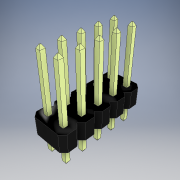
# Autodesk Inventor part: PinHeader-2x5-Male-NoCover
Saved by Autodesk Inventor 2018 (Build 220112000, 112)
## iProperties
Created: 2020-04-19
Part Number: PinHeader-2x5-Male-NoCover
Material: Všeobecné
Document SubType Name: Modeling
Designer: Jozko Mrkvicka
Density: 1 g/cm^3
Appearance: Výchozí
Author: Jozko Mrkvicka
Autodesk Inventor part; units mm, degrees
ref_plane "YZ Plane" through (0, 0, 0) normal (1, 0, 0) x (0, 1, 0)
ref_plane "XZ Plane" through (0, 0, 0) normal (0, 1, 0) x (-1, 0, 0)
ref_plane "XY Plane" through (0, 0, 0) normal (0, 0, 1) x (1, 0, 0)
sketch "Náčrt1" plane through (0, 0, 0) normal (0, 1, 0) x (-1, 0, 0)
  line L0 (0.635, 0) -> (4.445, 0)
  line L1 (4.445, -12.7) -> (0.635, -12.7)
  line L2 (0, -1.905) -> (0.635, -2.54)
  line L3 (0.635, -2.54) -> (0, -3.175)
  line L4 (0, -4.445) -> (0.635, -5.08)
  line L5 (0.635, -5.08) -> (0, -5.715)
  line L6 (0, -6.985) -> (0.635, -7.62)
  line L7 (0.635, -7.62) -> (0, -8.255)
  line L8 (0, -9.525) -> (0.635, -10.16)
  line L9 (0.635, -10.16) -> (0, -10.795)
  line L10 (0, -10.795) -> (0, -12.065)
  line L11 (0, -12.065) -> (0.635, -12.7)
  line L12 (0, -0.635) -> (0.635, 0)
  line L13 (4.445, 0) -> (5.08, -0.635)
  line L14 (5.08, -1.905) -> (4.445, -2.54)
  line L15 (4.445, -2.54) -> (5.08, -3.175)
  line L16 (5.08, -4.445) -> (4.445, -5.08)
  line L17 (4.445, -5.08) -> (5.08, -5.715)
  line L18 (5.08, -6.985) -> (4.445, -7.62)
  line L19 (4.445, -7.62) -> (5.08, -8.255)
  line L20 (5.08, -9.525) -> (4.445, -10.16)
  line L21 (4.445, -10.16) -> (5.08, -10.795)
  line L22 (5.08, -12.065) -> (4.445, -12.7)
  line L23 (0, -1.905) -> (0, -0.635)
  line L24 (0, -4.445) -> (0, -3.175)
  line L25 (0, -6.985) -> (0, -5.715)
  line L26 (0, -12.065) -> (0, -10.795)
  line L27 (0, -9.525) -> (0, -8.255)
  line L28 (5.08, -10.795) -> (5.08, -12.065)
  line L29 (5.08, -8.255) -> (5.08, -9.525)
  line L30 (5.08, -5.715) -> (5.08, -6.985)
  line L31 (5.08, -0.635) -> (5.08, -1.905)
  line L32 (5.08, -3.175) -> (5.08, -4.445)
  point P0 (0, 0)
  constraints: 66 end point, 26 parallel, 21 perpendicular, 1 horizontal
extrude "Vysunutí1" add sketch "Náčrt1" along normal blind 2.54
sketch "Náčrt2" plane through (0, 2.54, 0) normal (0, 1, 0) x (1, 0, 0)
  line L0 (-1.5875, 4.1275) -> (-1.5875, 3.4925)
  line L1 (-1.5875, 3.4925) -> (-0.9525, 3.4925)
  line L2 (-0.9525, 3.4925) -> (-0.9525, 4.1275)
  line L3 (-0.9525, 4.1275) -> (-1.5875, 4.1275)
  line L4 (-4.1275, 4.1275) -> (-4.1275, 3.4925)
  line L5 (-4.1275, 3.4925) -> (-3.4925, 3.4925)
  line L6 (-3.4925, 3.4925) -> (-3.4925, 4.1275)
  line L7 (-3.4925, 4.1275) -> (-4.1275, 4.1275)
  line L8 (-1.5875, 6.6675) -> (-1.5875, 6.0325)
  line L9 (-1.5875, 6.0325) -> (-0.9525, 6.0325)
  line L10 (-0.9525, 6.0325) -> (-0.9525, 6.6675)
  line L11 (-0.9525, 6.6675) -> (-1.5875, 6.6675)
  line L12 (-1.5875, 11.7475) -> (-1.5875, 11.1125)
  line L13 (-1.5875, 11.1125) -> (-0.9525, 11.1125)
  line L14 (-0.9525, 11.1125) -> (-0.9525, 11.7475)
  line L15 (-0.9525, 11.7475) -> (-1.5875, 11.7475)
  line L16 (-4.1275, 11.7475) -> (-4.1275, 11.1125)
  line L17 (-4.1275, 11.1125) -> (-3.4925, 11.1125)
  line L18 (-3.4925, 11.1125) -> (-3.4925, 11.7475)
  line L19 (-3.4925, 11.7475) -> (-4.1275, 11.7475)
  line L20 (-4.1275, 9.2075) -> (-4.1275, 8.5725)
  line L21 (-4.1275, 8.5725) -> (-3.4925, 8.5725)
  line L22 (-3.4925, 8.5725) -> (-3.4925, 9.2075)
  line L23 (-3.4925, 9.2075) -> (-4.1275, 9.2075)
  line L24 (-0.9525, 8.5725) -> (-0.9525, 9.2075)
  line L25 (-0.9525, 9.2075) -> (-1.5875, 9.2075)
  line L26 (-1.5875, 9.2075) -> (-1.5875, 8.5725)
  line L27 (-1.5875, 8.5725) -> (-0.9525, 8.5725)
  line L28 (-4.1275, 6.6675) -> (-4.1275, 6.0325)
  line L29 (-4.1275, 6.0325) -> (-3.4925, 6.0325)
  line L30 (-3.4925, 6.0325) -> (-3.4925, 6.6675)
  line L31 (-3.4925, 6.6675) -> (-4.1275, 6.6675)
  line L32 (-1.5875, 1.5875) -> (-1.5875, 0.9525)
  line L33 (-1.5875, 0.9525) -> (-0.9525, 0.9525)
  line L34 (-0.9525, 0.9525) -> (-0.9525, 1.5875)
  line L35 (-0.9525, 1.5875) -> (-1.5875, 1.5875)
  line L36 (-4.1275, 1.5875) -> (-4.1275, 0.9525)
  line L37 (-4.1275, 0.9525) -> (-3.4925, 0.9525)
  line L38 (-3.4925, 0.9525) -> (-3.4925, 1.5875)
  line L39 (-3.4925, 1.5875) -> (-4.1275, 1.5875)
  point P0 (0, 0)
  point P1 (-3.81, 1.27)
  constraints: 80 end point
extrude "Vysunutí2" add sketch "Náčrt2" along normal blind 8.255
sketch "Náčrt3" plane through (0, 0, 0) normal (0, -1, 0) x (1, 0, 0)
  line L0 (-1.5875, -1.5875) -> (-0.9525, -1.5875) projected
  line L1 (-0.9525, -1.5875) -> (-0.9525, -0.9525) projected
  line L2 (-0.9525, -0.9525) -> (-1.5875, -0.9525) projected
  line L3 (-1.5875, -0.9525) -> (-1.5875, -1.5875) projected
  line L4 (-1.5875, -6.6675) -> (-0.9525, -6.6675) projected
  line L5 (-0.9525, -6.6675) -> (-0.9525, -6.0325) projected
  line L6 (-0.9525, -6.0325) -> (-1.5875, -6.0325) projected
  line L7 (-1.5875, -6.0325) -> (-1.5875, -6.6675) projected
  line L8 (-1.5875, -4.1275) -> (-0.9525, -4.1275) projected
  line L9 (-0.9525, -4.1275) -> (-0.9525, -3.4925) projected
  line L10 (-0.9525, -3.4925) -> (-1.5875, -3.4925) projected
  line L11 (-1.5875, -3.4925) -> (-1.5875, -4.1275) projected
  line L12 (-4.1275, -9.2075) -> (-3.4925, -9.2075) projected
  line L13 (-3.4925, -9.2075) -> (-3.4925, -8.5725) projected
  line L14 (-3.4925, -8.5725) -> (-4.1275, -8.5725) projected
  line L15 (-4.1275, -8.5725) -> (-4.1275, -9.2075) projected
  line L16 (-1.5875, -11.7475) -> (-0.9525, -11.7475) projected
  line L17 (-0.9525, -11.7475) -> (-0.9525, -11.1125) projected
  line L18 (-0.9525, -11.1125) -> (-1.5875, -11.1125) projected
  line L19 (-1.5875, -11.1125) -> (-1.5875, -11.7475) projected
  line L20 (-4.1275, -11.7475) -> (-3.4925, -11.7475) projected
  line L21 (-3.4925, -11.7475) -> (-3.4925, -11.1125) projected
  line L22 (-3.4925, -11.1125) -> (-4.1275, -11.1125) projected
  line L23 (-4.1275, -11.1125) -> (-4.1275, -11.7475) projected
  line L24 (-0.9525, -9.2075) -> (-0.9525, -8.5725) projected
  line L25 (-0.9525, -8.5725) -> (-1.5875, -8.5725) projected
  line L26 (-1.5875, -8.5725) -> (-1.5875, -9.2075) projected
  line L27 (-1.5875, -9.2075) -> (-0.9525, -9.2075) projected
  line L28 (-4.1275, -4.1275) -> (-3.4925, -4.1275) projected
  line L29 (-3.4925, -4.1275) -> (-3.4925, -3.4925) projected
  line L30 (-3.4925, -3.4925) -> (-4.1275, -3.4925) projected
  line L31 (-4.1275, -3.4925) -> (-4.1275, -4.1275) projected
  line L32 (-4.1275, -6.6675) -> (-3.4925, -6.6675) projected
  line L33 (-3.4925, -6.6675) -> (-3.4925, -6.0325) projected
  line L34 (-3.4925, -6.0325) -> (-4.1275, -6.0325) projected
  line L35 (-4.1275, -6.0325) -> (-4.1275, -6.6675) projected
  line L36 (-4.1275, -1.5875) -> (-3.4925, -1.5875) projected
  line L37 (-3.4925, -1.5875) -> (-3.4925, -0.9525) projected
  line L38 (-3.4925, -0.9525) -> (-4.1275, -0.9525) projected
  line L39 (-4.1275, -0.9525) -> (-4.1275, -1.5875) projected
  line L40 (-5.08, -12.065) -> (-5.08, -10.795) projected
  line L41 (-5.08, -10.795) -> (-4.445, -10.16) projected
  line L42 (-4.445, -10.16) -> (-5.08, -9.525) projected
  line L43 (-5.08, -9.525) -> (-5.08, -8.255) projected
  line L44 (-5.08, -8.255) -> (-4.445, -7.62) projected
  line L45 (-4.445, -7.62) -> (-5.08, -6.985) projected
  line L46 (-5.08, -6.985) -> (-5.08, -5.715) projected
  line L47 (-5.08, -5.715) -> (-4.445, -5.08) projected
  line L48 (-4.445, -5.08) -> (-5.08, -4.445) projected
  line L49 (-5.08, -4.445) -> (-5.08, -3.175) projected
  line L50 (-5.08, -3.175) -> (-4.445, -2.54) projected
  line L51 (-4.445, -2.54) -> (-5.08, -1.905) projected
  line L52 (-5.08, -1.905) -> (-5.08, -0.635) projected
  line L53 (-5.08, -0.635) -> (-4.445, 0) projected
  line L54 (-4.445, 0) -> (-0.635, 0) projected
  line L55 (-0.635, 0) -> (0, -0.635) projected
  line L56 (0, -0.635) -> (0, -1.905) projected
  line L57 (0, -1.905) -> (-0.635, -2.54) projected
  line L58 (-0.635, -2.54) -> (0, -3.175) projected
  line L59 (0, -3.175) -> (0, -4.445) projected
  line L60 (0, -4.445) -> (-0.635, -5.08) projected
  line L61 (-0.635, -5.08) -> (0, -5.715) projected
  line L62 (0, -5.715) -> (0, -6.985) projected
  line L63 (0, -6.985) -> (-0.635, -7.62) projected
  line L64 (-0.635, -7.62) -> (0, -8.255) projected
  line L65 (0, -8.255) -> (0, -9.525) projected
  line L66 (0, -9.525) -> (-0.635, -10.16) projected
  line L67 (-0.635, -10.16) -> (0, -10.795) projected
  line L68 (0, -10.795) -> (0, -12.065) projected
  line L69 (0, -12.065) -> (-0.635, -12.7) projected
  line L70 (-0.635, -12.7) -> (-4.445, -12.7) projected
  line L71 (-4.445, -12.7) -> (-5.08, -12.065) projected
  point P0 (0, 0)
extrude "Vysunutí3" add sketch "Náčrt3" along normal blind 3.175 contours L3 L2 L1 L0 | L7 L6 L5 L4 | L11 L10 L9 L8 | L15 L14 L13 L12 | L19 L18 L17 L16 | L23 L22 L21 L20 | L27 L26 L25 L24 | L31 L30 L29 L28 | L35 L34 L33 L32 | L39 L38 L37 L36
chamfer "Zkosení1" distance 0.254 angle 60 4 edges at (-0.9525, 10.795, -1.27) (-1.27, 10.795, -0.9525) (-1.27, 10.795, -1.5875) (-1.5875, 10.795, -1.27) measured on face at (-1.3758, 10.795, -1.3758)
chamfer "Zkosení2" distance 0.254 angle 60 4 edges at (-3.4925, 10.795, -1.27) (-3.81, 10.795, -1.5875) (-3.81, 10.795, -0.9525) (-4.1275, 10.795, -1.27) measured on face at (-3.9158, 10.795, -1.3758)
chamfer "Zkosení3" distance 0.254 angle 60 4 edges at (-3.4925, 10.795, -3.81) (-3.81, 10.795, -4.1275) (-4.1275, 10.795, -3.81) (-3.81, 10.795, -3.4925) measured on face at (-3.9158, 10.795, -3.9158)
chamfer "Zkosení4" distance 0.254 angle 60 4 edges at (-1.5875, 10.795, -3.81) (-1.27, 10.795, -4.1275) (-0.9525, 10.795, -3.81) (-1.27, 10.795, -3.4925) measured on face at (-1.3758, 10.795, -3.9158)
chamfer "Zkosení5" distance 0.254 angle 60 4 edges at (-3.81, 10.795, -6.6675) (-4.1275, 10.795, -6.35) (-3.4925, 10.795, -6.35) (-3.81, 10.795, -6.0325) measured on face at (-3.9158, 10.795, -6.4558)
chamfer "Zkosení6" distance 0.254 angle 60 4 edges at (-1.27, 10.795, -6.6675) (-1.5875, 10.795, -6.35) (-0.9525, 10.795, -6.35) (-1.27, 10.795, -6.0325) measured on face at (-1.3758, 10.795, -6.4558)
chamfer "Zkosení7" distance 0.254 angle 60 4 edges at (-3.81, 10.795, -9.2075) (-4.1275, 10.795, -8.89) (-3.4925, 10.795, -8.89) (-3.81, 10.795, -8.5725) measured on face at (-3.9158, 10.795, -8.9958)
chamfer "Zkosení8" distance 0.254 angle 60 4 edges at (-0.9525, 10.795, -8.89) (-1.27, 10.795, -9.2075) (-1.5875, 10.795, -8.89) (-1.27, 10.795, -8.5725) measured on face at (-1.3758, 10.795, -8.9958)
chamfer "Zkosení9" distance 0.254 angle 60 4 edges at (-3.4925, 10.795, -11.43) (-3.81, 10.795, -11.7475) (-4.1275, 10.795, -11.43) (-3.81, 10.795, -11.1125) measured on face at (-3.9158, 10.795, -11.5358)
chamfer "Zkosení10" distance 0.254 angle 60 4 edges at (-1.5875, 10.795, -11.43) (-1.27, 10.795, -11.7475) (-0.9525, 10.795, -11.43) (-1.27, 10.795, -11.1125) measured on face at (-1.3758, 10.795, -11.5358)
chamfer "Zkosení11" distance 0.254 angle 60 4 edges at (-4.1275, -3.175, -11.43) (-3.81, -3.175, -11.1125) (-3.4925, -3.175, -11.43) (-3.81, -3.175, -11.7475) measured on face at (-3.9158, -3.175, -11.3242)
chamfer "Zkosení12" distance 0.254 angle 60 4 edges at (-1.5875, -3.175, -11.43) (-1.27, -3.175, -11.1125) (-0.9525, -3.175, -11.43) (-1.27, -3.175, -11.7475) measured on face at (-1.3758, -3.175, -11.3242)
chamfer "Zkosení13" distance 0.254 angle 60 4 edges at (-4.1275, -3.175, -8.89) (-3.81, -3.175, -8.5725) (-3.4925, -3.175, -8.89) (-3.81, -3.175, -9.2075) measured on face at (-3.9158, -3.175, -8.7842)
chamfer "Zkosení14" distance 0.254 angle 60 4 edges at (-1.5875, -3.175, -8.89) (-1.27, -3.175, -8.5725) (-0.9525, -3.175, -8.89) (-1.27, -3.175, -9.2075) measured on face at (-1.1642, -3.175, -8.9958)
chamfer "Zkosení15" distance 0.254 angle 60 4 edges at (-4.1275, -3.175, -6.35) (-3.81, -3.175, -6.6675) (-3.81, -3.175, -6.0325) (-3.4925, -3.175, -6.35) measured on face at (-3.9158, -3.175, -6.2442)
chamfer "Zkosení16" distance 0.254 angle 60 4 edges at (-1.5875, -3.175, -6.35) (-1.27, -3.175, -6.0325) (-0.9525, -3.175, -6.35) (-1.27, -3.175, -6.6675) measured on face at (-1.3758, -3.175, -6.2442)
chamfer "Zkosení17" distance 0.254 angle 60 4 edges at (-4.1275, -3.175, -3.81) (-3.81, -3.175, -3.4925) (-3.4925, -3.175, -3.81) (-3.81, -3.175, -4.1275) measured on face at (-3.9158, -3.175, -3.7042)
chamfer "Zkosení18" distance 0.254 angle 60 4 edges at (-1.5875, -3.175, -3.81) (-0.9525, -3.175, -3.81) (-1.27, -3.175, -3.4925) (-1.27, -3.175, -4.1275) measured on face at (-1.3758, -3.175, -3.7042)
chamfer "Zkosení19" distance 0.254 angle 60 4 edges at (-4.1275, -3.175, -1.27) (-3.81, -3.175, -0.9525) (-3.4925, -3.175, -1.27) (-3.81, -3.175, -1.5875) measured on face at (-3.9158, -3.175, -1.1642)
chamfer "Zkosení20" distance 0.254 angle 60 4 edges at (-1.5875, -3.175, -1.27) (-1.27, -3.175, -0.9525) (-0.9525, -3.175, -1.27) (-1.27, -3.175, -1.5875) measured on face at (-1.3758, -3.175, -1.1642)
